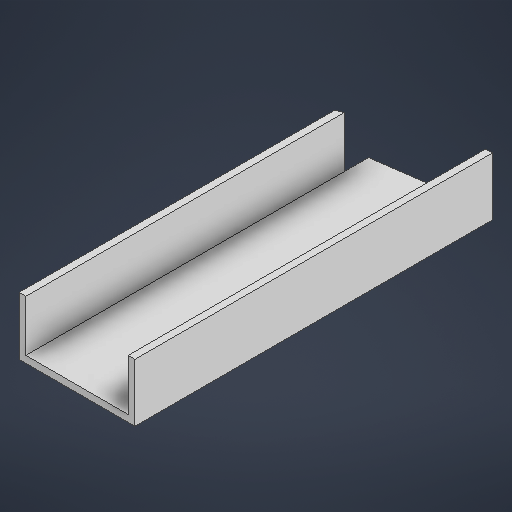
# Autodesk Inventor part: outslideleft
Saved by Autodesk Inventor 2026.2 (Build 302298000, 298)
## iProperties
Created: 2026-02-23
Part Number: outslideleft
Material: Generic
Document SubType Name: Sheet Metal
Designer: danda
Density: 1 g/cm^3
Sheet Metal Rule: Default_mm
Appearance: Default
Author: danda
Autodesk Inventor part; units mm, degrees
ref_plane "YZ Plane" through (0, 0, 0) normal (1, 0, 0) x (0, 1, 0)
ref_plane "XZ Plane" through (0, 0, 0) normal (0, 1, 0) x (-1, 0, 0)
ref_plane "XY Plane" through (0, 0, 0) normal (0, 0, 1) x (1, 0, 0)
sketch "Sketch1" plane through (0, 0, 0) normal (0, 0, 1) x (1, 0, 0)
  line L0 (10.7104, 9.7791) -> (40.7104, 9.7791)
  line L1 (40.7104, 9.7791) -> (40.7104, 24.7791)
  line L2 (10.7104, 9.7791) -> (10.7104, 24.7791)
  line L3 (8.7104, 24.7791) -> (8.7104, 7.7791)
  line L4 (8.7104, 7.7791) -> (42.7104, 7.7791)
  line L5 (42.7104, 7.7791) -> (42.7104, 24.7791)
  line L6 (8.7104, 24.7791) -> (10.7104, 24.7791)
  line L7 (40.7104, 24.7791) -> (42.7104, 24.7791)
  point P0 (0, 0)
  dimension "d0" = 30
  dimension "d1" = 15
  dimension "d2" = 15
  dimension "d3" = 2
  constraints: 16 end point, 3 horizontal, 2 perpendicular, 1 vertical, 2 other
  measures "d0" distance of L0.start L0.end
  measures "d1" distance of L0.end L1.end
  measures "d2" distance of L0.start L2.end
  measures "d3" distance between parallel lines of L2 L3
extrude "Extrusion1" add sketch "Sketch1" along normal blind 100 and the other way blind 5
sketch "Sketch3" plane through (10.7104, 9.7791, 100) normal (0, 1, 0) x (1, 0, 0)
  line L0 (-2, 105) -> (-2, 0) projected
  line L1 (-2, 92.625) -> (-2, 105)
  line L2 (30, 105) -> (32, 105) projected
  line L3 (32, 105) -> (-2, 92.625)
  line L4 (-2, 105) -> (-2, 92.625)
  line L5 (-2, 105) -> (32, 105)
  line L6 (0, 105) -> (0, 0) projected
  line L7 (0, 93.353) -> (0, 105)
  line L8 (32, 105) -> (-2, 100.2216)
  line L9 (32, 105) -> (66.3341, 105) construction
  line L10 (-2, 100.2216) -> (-2, 105)
  point P0 (-10.7104, 100)
  point P1 (-2, 100.2216)
  point P2 (0, 100.5027)
  dimension "d15" = 20
  dimension "d16" = 172
  constraints: 16 end point, 4 point on line, 3 collinear, 1 equal length, 1 horizontal, 1 perpendicular
  measures "d15" angle of L3 L5
  measures "d16" angle of L8 L9
extrude "Extrusion4" cut sketch "Sketch3" along normal through all both and the other way through all contours L5 L6 L8 L0 | L5 L2 L8 L6
extrude "Extrusion5" cut sketch "Sketch3" along normal through all both and the other way through all contours L8 L6 L3 L0
equation "\"BendRadius\" = Thickness"
equation "\"BendReliefWidth\" = Thickness"
equation "\"BendReliefDepth\" = 0.5 * Thickness"
equation "\"CornerReliefSize\" = 4 * Thickness"
equation "\"MinimumRemnant\" = 2 * Thickness"
equation "\"TransitionRadius\" = BendRadius"
equation "\"JacobiRadiusSize\" = BendRadius"
equation "\"GapSize\" = Thickness"
equation "\"Thickness\" = 0.5"
body "Solid1"
